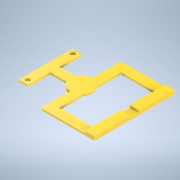
# Autodesk Inventor part: BaseGripper
Saved by Autodesk Inventor 2021 (Build 250183000, 183)
## iProperties
Created: 2022-11-01
Part Number: BaseGripper
Material: Generic
Document SubType Name: Modeling
Designer: USUARIO
Density: 1 g/cm^3
Appearance: Glossy - Gold
Author: USUARIO
Autodesk Inventor part; units mm, degrees
ref_plane "YZ Plane" through (0, 0, 0) normal (1, 0, 0) x (0, 1, 0)
ref_plane "XZ Plane" through (0, 0, 0) normal (0, 1, 0) x (-1, 0, 0)
ref_plane "XY Plane" through (0, 0, 0) normal (0, 0, 1) x (1, 0, 0)
sketch "Sketch1" plane through (0, 0, 0) normal (0, 1, 0) x (-1, 0, 0)
  line L0 (-40, 70) -> (40, 70)
  line L1 (40, 70) -> (40, -70)
  line L2 (40, -70) -> (-40, -70)
  line L3 (-40, -70) -> (-40, 70)
  line L4 (-40, 70) -> (40, -70) construction
  line L5 (40, 70) -> (-40, -70) construction
  line L6 (60, -90) -> (60, 90)
  line L7 (60, 90) -> (-60, 90)
  line L8 (-60, 90) -> (-60, -90)
  line L9 (-60, -90) -> (60, -90)
  line L10 (120, 10) -> (60, 10)
  line L11 (60, 10) -> (60, -10)
  line L12 (60, -10) -> (120, -10)
  line L13 (120, -10) -> (120, 10)
  line L14 (120, 10) -> (60, -10) construction
  line L15 (60, 10) -> (120, -10) construction
  line L16 (140, -60) -> (120, -60)
  line L17 (120, -60) -> (120, 60)
  line L18 (120, 60) -> (140, 60)
  line L19 (140, 60) -> (140, -60)
  line L20 (140, -60) -> (120, 60) construction
  line L21 (120, -60) -> (140, 60) construction
  line L22 (180, 0) -> (-100, 0) projected
  circle A0 centre (60, 0) radius 25
  circle A1 centre (130, 51) radius 5
  circle A2 centre (130, -51) radius 5
  point P0 (0, 0)
  point P1 (90, 0)
  point P2 (130, 0)
  point P3 (90, 0)
  point P4 (130, 0)
  point P5 (60, 25)
  point P6 (60, -25)
  point P7 (82.9129, -10)
  point P8 (120, 10)
  point P9 (82.9129, 10)
  point P10 (40, -15)
  point P11 (40, 15)
  dimension "d0" = 20
  dimension "d1" = 20
  dimension "d2" = 20
  dimension "d3" = 200
  dimension "d4" = 120
  dimension "d5" = 120
  dimension "d6" = 180
  dimension "d7" = 50
  dimension "d8" = 10
  dimension "d9" = 9
  dimension "d10" = 10
  dimension "d11" = 9
  dimension "d12" = 10
  dimension "d13" = 10
  constraints: 44 end point, 9 midpoint, 8 parallel, 5 point on line, 4 perpendicular, 3 centre point, 3 horizontal, 3 other
  measures "d0" distance between parallel lines of L1 L6
  measures "d1" distance between parallel lines of L10 L12
  measures "d2" distance between parallel lines of L17 L19
  measures "d3" distance between parallel lines of L8 L19
  measures "d4" distance of L6.end L7.end
  measures "d5" distance of L18.end L16.start
  measures "d6" distance of L7.end L8.end
  measures "d7" diameter of A0
  measures "d8" distance from line of L19 A2.centre
  measures "d9" distance from line of L16 A2.centre
  measures "d10" diameter of A2
  measures "d11" distance from line of L18 A1.centre
  measures "d12" diameter of A1
  measures "d13" distance from line of L19 A1.centre
extrude "Extrusion1" add sketch "Sketch1" along normal blind 5 contours L3 L22 L8 L7 L6 A0 L1 L0 | L3 L2 L1 A0 L6 L9 L8 L22 | A0 L6 L22 L1 | L1 L22 A0 | L22 L1 A0 | L22 L6 A0 L1 | A0 L10 L6 | L22 A0 L12 L6 | L6 L10 A0 L22 | L10 L13 L22 A0 | L6 L12 A0 | L22 L13 L12 A0 | L17 L18 L19 L22 L13 | L22 L19 L16 L17 L13
sketch "Sketch2" plane through (0, 5, 0) normal (0, 1, 0) x (1, 0, 0)
  line L0 (-60, -90) -> (60, -90) projected
  line L1 (60, -90) -> (60, 90) projected
  line L2 (60, 90) -> (-60, 90) projected
  line L3 (-60, 90) -> (-60, 25) projected
  arc A0 (-60, 25) -> (-82.9129, 10) centre (-60, 0) ccw projected
  line L4 (-82.9129, 10) -> (-120, 10) projected
  line L5 (-120, 10) -> (-120, 60) projected
  line L6 (-120, 60) -> (-140, 60) projected
  line L7 (-140, 60) -> (-140, -60) projected
  line L8 (-140, -60) -> (-120, -60) projected
  line L9 (-120, -60) -> (-120, -10) projected
  line L10 (-120, -10) -> (-82.9129, -10) projected
  arc A1 (-82.9129, -10) -> (-60, -25) centre (-60, 0) ccw projected
  line L11 (-60, -25) -> (-60, -90) projected
  circle A2 centre (-130, 51) radius 5 projected
  circle A3 centre (-130, -51) radius 5 projected
  arc A4 (-40, -15) -> (-40, 15) centre (-60, 0) ccw projected
  line L12 (-40, 15) -> (-40, 70) projected
  line L13 (-40, 70) -> (40, 70) projected
  line L14 (40, 70) -> (40, -70) projected
  line L15 (40, -70) -> (-40, -70) projected
  line L16 (-40, -70) -> (-40, -15) projected
  line L17 (-60, -90) -> (60, -90) projected
  line L18 (60, -90) -> (40, -90)
  line L19 (40, -90) -> (40, 90)
  line L20 (40, 90) -> (60, 90)
  line L21 (60, 90) -> (60, -90)
  line L22 (40, 70) -> (40, -70) projected
  line L23 (60, -90) -> (60, 90) projected
  line L24 (40, -10) -> (60, -10)
  line L25 (60, -10) -> (60, 10)
  line L26 (60, 10) -> (40, 10)
  line L27 (40, 10) -> (40, -10)
  point P0 (0, 0)
  point P1 (40, 10)
  point P2 (60, 10)
  point P3 (60, -10)
  point P4 (40, -10)
  dimension "d16" = 20
  dimension "d17" = 10
  constraints: 16 end point, 4 parallel, 3 point on line, 2 horizontal, 2 perpendicular
  measures "d16" distance between parallel lines of L24 L26
  measures "d17" distance from line of point (0, 0) L26
extrude "Extrusion2" add sketch "Sketch2" along normal blind 5 contours L19 L14 L24 L1 L0 | L26 L14 L19 L2 L1
equation "\"d0\" = AnEsl"
equation "\"d1\" = AnEsl"
equation "\"d2\" = AnEsl"
equation "\"d6\" = 1.5 * d5"
equation "\"d7\" = DV"
equation "\"d8\" = 0.5 * d2"
equation "\"d11\" = d9"
equation "\"d12\" = d10"
equation "\"d13\" = d8"
equation "\"d17\" = 0.5 * d16"
equation "\"DV\" = 50"
equation "\"AnEsl\" = 20"
body "Solid1"
